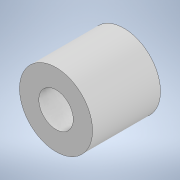
# Autodesk Inventor part: bearing L30 d32.25
Saved by Autodesk Inventor 2021 (Build 250183000, 183)
## iProperties
Created: 2021-04-14
Part Number: bearing L30 d32.25
Material: Generic
Document SubType Name: Modeling
Designer: Olivi
Density: 1 g/cm^3
Appearance: Default
Author: Olivi
Autodesk Inventor part; units mm, degrees
ref_plane "YZ Plane" through (0, 0, 0) normal (1, 0, 0) x (0, 1, 0)
ref_plane "XZ Plane" through (0, 0, 0) normal (0, 1, 0) x (-1, 0, 0)
ref_plane "XY Plane" through (0, 0, 0) normal (0, 0, 1) x (1, 0, 0)
sketch "Sketch1" plane through (0, 0, 0) normal (0, 0, 1) x (1, 0, 0)
  circle A0 centre (0, 0) radius 16.125
  circle A1 centre (0, 0) radius 7.6
  dimension "d0" = 32.25
  dimension "d1" = 15.2
  constraints: 2 centre point, 2 coincident
  measures "d0" diameter of A0
  measures "d1" diameter of A1
extrude "Extrusion1" add sketch "Sketch1" along normal blind 30
body "Solid1"
